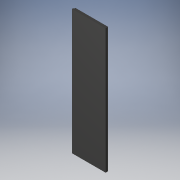
# Autodesk Inventor part: BA09
Saved by Autodesk Inventor 2017 (Build 210142000, 142)
## iProperties
Created: 2018-10-18
Part Number: BA09
Material: ABS Plastic
Document SubType Name: Modeling
Designer: Dell
Density: 1.06 g/cm^3
Appearance: Smooth - Black
Author: Dell
Autodesk Inventor part; units mm, degrees
ref_plane "YZ Plane" through (0, 0, 0) normal (1, 0, 0) x (0, 1, 0)
ref_plane "XZ Plane" through (0, 0, 0) normal (0, 1, 0) x (-1, 0, 0)
ref_plane "XY Plane" through (0, 0, 0) normal (0, 0, 1) x (1, 0, 0)
sketch "Sketch1" plane through (0, 0, 0) normal (0, 0, 1) x (1, 0, 0)
  line L0 (0, 0) -> (95.25, 0)
  line L1 (95.25, 0) -> (95.25, 355.6)
  line L2 (95.25, 355.6) -> (0, 355.6)
  line L3 (0, 355.6) -> (0, 0)
  dimension "d0" = 95.25
  dimension "d1" = 355.6
  constraints: 8 end point, 2 parallel, 1 horizontal, 1 perpendicular
  measures "d0" distance of L2.end L1.end
  measures "d1" distance of L0.end L1.end
extrude "Extrusion1" add sketch "Sketch1" along normal blind 6.35
sketch "Sketch2" plane through (0, 355.6, 0) normal (0, 1, 0) x (1, 0, 0)
  line L0 (0, -6.35) -> (95.25, -6.35) projected
  line L1 (0, -6.35) -> (3.6662, 0)
  line L2 (0, 0) -> (95.25, 0) projected
  line L3 (0, 0) -> (0, -6.35)
  line L4 (3.6662, 0) -> (0, 0)
  dimension "d4" = 30
  constraints: 6 end point, 1 perpendicular, 1 point on line, 1 vertical
  measures "d4" angle of L3 L1
extrude "Extrusion2" cut sketch "Sketch2" against normal blind 355.6
body "Solid1"
